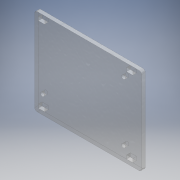
# Autodesk Inventor part: BBGW Case Bottom
Saved by Autodesk Inventor 2016 (Build 200138000, 138)
## iProperties
Created: 2016-06-26
Part Number: BBGW Case Bottom
Material: Acrylic, Clear
Document SubType Name: Modeling
Designer: Jacob
Density: 1.19 g/cm^3
Appearance: Transparent - Clear
Author: Jacob
Autodesk Inventor part; units mm, degrees
(part 1 of 2)
ref_plane "YZ Plane" through (0, 0, 0) normal (1, 0, 0) x (0, 1, 0)
ref_plane "XZ Plane" through (0, 0, 0) normal (0, 1, 0) x (-1, 0, 0)
ref_plane "XY Plane" through (0, 0, 0) normal (0, 0, 1) x (1, 0, 0)
sketch "Sketch1" plane through (0, 0, 0) normal (0, 1, 0) x (-1, 0, 0)
  line L0 (76.6427, 130.7252) -> (76.6428, 139.3252)
  spline S0 degree 3 poles (76.6428, 139.3252) (76.6428, 140.4298) (75.7473, 141.3252) (74.6428, 141.3252) knots 0 0 0 0 1 1 1 1
  line L1 (76.6428, 139.3252) -> (76.6428, 140.4298) construction
  line L2 (76.6428, 140.4298) -> (75.7473, 141.3252) construction
  line L3 (75.7473, 141.3252) -> (74.6428, 141.3252) construction
  line L4 (74.6428, 141.3252) -> (73.6427, 141.3252)
  line L5 (73.6427, 141.3252) -> (73.6427, 143.3252)
  line L6 (73.6427, 143.3252) -> (73.6422, 143.3593)
  line L7 (73.6422, 143.3593) -> (73.6404, 143.3934)
  line L8 (73.6404, 143.3934) -> (73.6375, 143.4275)
  line L9 (73.6375, 143.4275) -> (73.6334, 143.4614)
  line L10 (73.6334, 143.4614) -> (73.6282, 143.4951)
  line L11 (73.6282, 143.4951) -> (73.6218, 143.5287)
  line L12 (73.6218, 143.5287) -> (73.6143, 143.562)
  line L13 (73.6143, 143.562) -> (73.6057, 143.595)
  line L14 (73.6057, 143.595) -> (73.5959, 143.6277)
  line L15 (73.5959, 143.6277) -> (73.585, 143.6601)
  line L16 (73.585, 143.6601) -> (73.573, 143.6921)
  line L17 (73.573, 143.6921) -> (73.56, 143.7236)
  line L18 (73.56, 143.7236) -> (73.5458, 143.7547)
  line L19 (73.5458, 143.7547) -> (73.5306, 143.7853)
  line L20 (73.5306, 143.7853) -> (73.5144, 143.8153)
  line L21 (73.5144, 143.8153) -> (73.4972, 143.8448)
  line L22 (73.4972, 143.8448) -> (73.4789, 143.8737)
  line L23 (73.4789, 143.8737) -> (73.4597, 143.9019)
  line L24 (73.4597, 143.9019) -> (73.4396, 143.9294)
  line L25 (73.4396, 143.9294) -> (73.4185, 143.9563)
  line L26 (73.4185, 143.9563) -> (73.3965, 143.9824)
  line L27 (73.3965, 143.9824) -> (73.3736, 144.0078)
  line L28 (73.3736, 144.0078) -> (73.3499, 144.0323)
  line L29 (73.3499, 144.0323) -> (73.3253, 144.056)
  line L30 (73.3253, 144.056) -> (73.3, 144.0789)
  line L31 (73.3, 144.0789) -> (73.2738, 144.1009)
  line L32 (73.2738, 144.1009) -> (73.247, 144.122)
  line L33 (73.247, 144.122) -> (73.2194, 144.1422)
  line L34 (73.2194, 144.1422) -> (73.1912, 144.1614)
  line L35 (73.1912, 144.1614) -> (73.1623, 144.1796)
  line L36 (73.1623, 144.1796) -> (73.1329, 144.1969)
  line L37 (73.1329, 144.1969) -> (73.1028, 144.2131)
  line L38 (73.1028, 144.2131) -> (73.0722, 144.2283)
  line L39 (73.0722, 144.2283) -> (73.0412, 144.2424)
  line L40 (73.0412, 144.2424) -> (73.0096, 144.2555)
  line L41 (73.0096, 144.2555) -> (72.9776, 144.2675)
  line L42 (72.9776, 144.2675) -> (72.9453, 144.2783)
  line L43 (72.9453, 144.2783) -> (72.9125, 144.2881)
  line L44 (72.9125, 144.2881) -> (72.8795, 144.2968)
  line L45 (72.8795, 144.2968) -> (72.8462, 144.3043)
  line L46 (72.8462, 144.3043) -> (72.8127, 144.3107)
  line L47 (72.8127, 144.3107) -> (72.7789, 144.3159)
  line L48 (72.7789, 144.3159) -> (72.745, 144.32)
  line L49 (72.745, 144.32) -> (72.711, 144.3229)
  line L50 (72.711, 144.3229) -> (72.6769, 144.3246)
  line L51 (72.6769, 144.3246) -> (72.6428, 144.3252)
  line L52 (72.6428, 144.3252) -> (69.6427, 144.3252)
  line L53 (69.6427, 144.3252) -> (69.6086, 144.3246)
  line L54 (69.6086, 144.3246) -> (69.5745, 144.3229)
  line L55 (69.5745, 144.3229) -> (69.5405, 144.32)
  line L56 (69.5405, 144.32) -> (69.5066, 144.3159)
  line L57 (69.5066, 144.3159) -> (69.4728, 144.3107)
  line L58 (69.4728, 144.3107) -> (69.4393, 144.3043)
  line L59 (69.4393, 144.3043) -> (69.406, 144.2968)
  line L60 (69.406, 144.2968) -> (69.373, 144.2881)
  line L61 (69.373, 144.2881) -> (69.3402, 144.2783)
  line L62 (69.3402, 144.2783) -> (69.3079, 144.2675)
  line L63 (69.3079, 144.2675) -> (69.2759, 144.2555)
  line L64 (69.2759, 144.2555) -> (69.2443, 144.2424)
  line L65 (69.2443, 144.2424) -> (69.2133, 144.2283)
  line L66 (69.2133, 144.2283) -> (69.1827, 144.2131)
  line L67 (69.1827, 144.2131) -> (69.1526, 144.1969)
  line L68 (69.1526, 144.1969) -> (69.1232, 144.1796)
  line L69 (69.1232, 144.1796) -> (69.0943, 144.1614)
  line L70 (69.0943, 144.1614) -> (69.0661, 144.1422)
  line L71 (69.0661, 144.1422) -> (69.0385, 144.122)
  line L72 (69.0385, 144.122) -> (69.0117, 144.1009)
  line L73 (69.0117, 144.1009) -> (68.9855, 144.0789)
  line L74 (68.9855, 144.0789) -> (68.9602, 144.056)
  line L75 (68.9602, 144.056) -> (68.9356, 144.0323)
  line L76 (68.9356, 144.0323) -> (68.9119, 144.0078)
  line L77 (68.9119, 144.0078) -> (68.889, 143.9824)
  line L78 (68.889, 143.9824) -> (68.867, 143.9563)
  line L79 (68.867, 143.9563) -> (68.8459, 143.9294)
  line L80 (68.8459, 143.9294) -> (68.8258, 143.9019)
  line L81 (68.8258, 143.9019) -> (68.8066, 143.8737)
  line L82 (68.8066, 143.8737) -> (68.7883, 143.8448)
  line L83 (68.7883, 143.8448) -> (68.7711, 143.8153)
  line L84 (68.7711, 143.8153) -> (68.7549, 143.7853)
  line L85 (68.7549, 143.7853) -> (68.7397, 143.7547)
  line L86 (68.7397, 143.7547) -> (68.7255, 143.7236)
  line L87 (68.7255, 143.7236) -> (68.7125, 143.6921)
  line L88 (68.7125, 143.6921) -> (68.7005, 143.6601)
  line L89 (68.7005, 143.6601) -> (68.6896, 143.6277)
  line L90 (68.6896, 143.6277) -> (68.6798, 143.595)
  line L91 (68.6798, 143.595) -> (68.6712, 143.562)
  line L92 (68.6712, 143.562) -> (68.6637, 143.5287)
  line L93 (68.6637, 143.5287) -> (68.6573, 143.4951)
  line L94 (68.6573, 143.4951) -> (68.6521, 143.4614)
  line L95 (68.6521, 143.4614) -> (68.648, 143.4275)
  line L96 (68.648, 143.4275) -> (68.6451, 143.3934)
  line L97 (68.6451, 143.3934) -> (68.6433, 143.3593)
  line L98 (68.6433, 143.3593) -> (68.6427, 143.3252)
  line L99 (68.6427, 143.3252) -> (68.6427, 141.3252)
  line L100 (68.6427, 141.3252) -> (1.8263, 141.3252)
  line L101 (1.8263, 141.3252) -> (1.8263, 143.3252)
  line L102 (1.8263, 143.3252) -> (1.8258, 143.3593)
  line L103 (1.8258, 143.3593) -> (1.824, 143.3934)
  line L104 (1.824, 143.3934) -> (1.8211, 143.4275)
  line L105 (1.8211, 143.4275) -> (1.817, 143.4614)
  line L106 (1.817, 143.4614) -> (1.8118, 143.4951)
  line L107 (1.8118, 143.4951) -> (1.8054, 143.5287)
  line L108 (1.8054, 143.5287) -> (1.7979, 143.562)
  line L109 (1.7979, 143.562) -> (1.7893, 143.595)
  line L110 (1.7893, 143.595) -> (1.7795, 143.6277)
  line L111 (1.7795, 143.6277) -> (1.7686, 143.6601)
  line L112 (1.7686, 143.6601) -> (1.7566, 143.6921)
  line L113 (1.7566, 143.6921) -> (1.7436, 143.7236)
  line L114 (1.7436, 143.7236) -> (1.7294, 143.7547)
  line L115 (1.7294, 143.7547) -> (1.7142, 143.7853)
  line L116 (1.7142, 143.7853) -> (1.698, 143.8153)
  line L117 (1.698, 143.8153) -> (1.6808, 143.8448)
  line L118 (1.6808, 143.8448) -> (1.6625, 143.8737)
  line L119 (1.6625, 143.8737) -> (1.6433, 143.9019)
  line L120 (1.6433, 143.9019) -> (1.6231, 143.9294)
  line L121 (1.6231, 143.9294) -> (1.6021, 143.9563)
  line L122 (1.6021, 143.9563) -> (1.5801, 143.9824)
  line L123 (1.5801, 143.9824) -> (1.5572, 144.0078)
  line L124 (1.5572, 144.0078) -> (1.5334, 144.0323)
  line L125 (1.5334, 144.0323) -> (1.5089, 144.056)
  line L126 (1.5089, 144.056) -> (1.4835, 144.0789)
  line L127 (1.4835, 144.0789) -> (1.4574, 144.1009)
  line L128 (1.4574, 144.1009) -> (1.4306, 144.122)
  line L129 (1.4306, 144.122) -> (1.403, 144.1422)
  line L130 (1.403, 144.1422) -> (1.3748, 144.1614)
  line L131 (1.3748, 144.1614) -> (1.3459, 144.1796)
  line L132 (1.3459, 144.1796) -> (1.3164, 144.1969)
  line L133 (1.3164, 144.1969) -> (1.2864, 144.2131)
  line L134 (1.2864, 144.2131) -> (1.2558, 144.2283)
  line L135 (1.2558, 144.2283) -> (1.2247, 144.2424)
  line L136 (1.2247, 144.2424) -> (1.1932, 144.2555)
  line L137 (1.1932, 144.2555) -> (1.1612, 144.2675)
  line L138 (1.1612, 144.2675) -> (1.1289, 144.2783)
  line L139 (1.1289, 144.2783) -> (1.0961, 144.2881)
  line L140 (1.0961, 144.2881) -> (1.0631, 144.2968)
  line L141 (1.0631, 144.2968) -> (1.0298, 144.3043)
  line L142 (1.0298, 144.3043) -> (0.9962, 144.3107)
  line L143 (0.9962, 144.3107) -> (0.9625, 144.3159)
  line L144 (0.9625, 144.3159) -> (0.9286, 144.32)
  line L145 (0.9286, 144.32) -> (0.8946, 144.3229)
  line L146 (0.8946, 144.3229) -> (0.8605, 144.3246)
  line L147 (0.8605, 144.3246) -> (0.8263, 144.3252)
  line L148 (0.8263, 144.3252) -> (-2.1737, 144.3252)
  line L149 (-2.1737, 144.3252) -> (-2.2078, 144.3246)
  line L150 (-2.2078, 144.3246) -> (-2.2419, 144.3229)
  line L151 (-2.2419, 144.3229) -> (-2.2759, 144.32)
  line L152 (-2.2759, 144.32) -> (-2.3098, 144.3159)
  line L153 (-2.3098, 144.3159) -> (-2.3436, 144.3107)
  line L154 (-2.3436, 144.3107) -> (-2.3771, 144.3043)
  line L155 (-2.3771, 144.3043) -> (-2.4104, 144.2968)
  line L156 (-2.4104, 144.2968) -> (-2.4435, 144.2881)
  line L157 (-2.4435, 144.2881) -> (-2.4762, 144.2783)
  line L158 (-2.4762, 144.2783) -> (-2.5085, 144.2675)
  line L159 (-2.5085, 144.2675) -> (-2.5405, 144.2555)
  line L160 (-2.5405, 144.2555) -> (-2.5721, 144.2424)
  line L161 (-2.5721, 144.2424) -> (-2.6031, 144.2283)
  line L162 (-2.6031, 144.2283) -> (-2.6337, 144.2131)
  line L163 (-2.6337, 144.2131) -> (-2.6638, 144.1969)
  line L164 (-2.6638, 144.1969) -> (-2.6932, 144.1796)
  line L165 (-2.6932, 144.1796) -> (-2.7221, 144.1614)
  line L166 (-2.7221, 144.1614) -> (-2.7503, 144.1422)
  line L167 (-2.7503, 144.1422) -> (-2.7779, 144.122)
  line L168 (-2.7779, 144.122) -> (-2.8047, 144.1009)
  line L169 (-2.8047, 144.1009) -> (-2.8309, 144.0789)
  line L170 (-2.8309, 144.0789) -> (-2.8562, 144.056)
  line L171 (-2.8562, 144.056) -> (-2.8808, 144.0323)
  line L172 (-2.8808, 144.0323) -> (-2.9045, 144.0078)
  line L173 (-2.9045, 144.0078) -> (-2.9274, 143.9824)
  line L174 (-2.9274, 143.9824) -> (-2.9494, 143.9563)
  line L175 (-2.9494, 143.9563) -> (-2.9705, 143.9294)
  line L176 (-2.9705, 143.9294) -> (-2.9906, 143.9019)
  line L177 (-2.9906, 143.9019) -> (-3.0098, 143.8737)
  line L178 (-3.0098, 143.8737) -> (-3.0281, 143.8448)
  line L179 (-3.0281, 143.8448) -> (-3.0453, 143.8153)
  line L180 (-3.0453, 143.8153) -> (-3.0615, 143.7853)
  line L181 (-3.0615, 143.7853) -> (-3.0767, 143.7547)
  line L182 (-3.0767, 143.7547) -> (-3.0909, 143.7236)
  line L183 (-3.0909, 143.7236) -> (-3.1039, 143.6921)
  line L184 (-3.1039, 143.6921) -> (-3.1159, 143.6601)
  line L185 (-3.1159, 143.6601) -> (-3.1268, 143.6277)
  line L186 (-3.1268, 143.6277) -> (-3.1366, 143.595)
  line L187 (-3.1366, 143.595) -> (-3.1452, 143.562)
  line L188 (-3.1452, 143.562) -> (-3.1527, 143.5287)
  line L189 (-3.1527, 143.5287) -> (-3.1591, 143.4951)
  line L190 (-3.1591, 143.4951) -> (-3.1643, 143.4614)
  line L191 (-3.1643, 143.4614) -> (-3.1684, 143.4275)
  line L192 (-3.1684, 143.4275) -> (-3.1713, 143.3934)
  line L193 (-3.1713, 143.3934) -> (-3.1731, 143.3593)
  line L194 (-3.1731, 143.3593) -> (-3.1737, 143.3252)
  line L195 (-3.1737, 143.3252) -> (-3.1737, 141.3252)
  line L196 (-3.1737, 141.3252) -> (-8.3571, 141.3252)
  spline S1 degree 3 poles (-8.3571, 141.3252) (-8.8876, 141.3252) (-9.3963, 141.1145) (-9.7714, 140.7394) knots 0 0 0 0 0.5 0.5 0.5 0.5
  line L197 (-8.3571, 141.3252) -> (-8.8876, 141.3252) construction
  line L198 (-8.8876, 141.3252) -> (-9.3963, 141.1145) construction
  line L199 (-9.3963, 141.1145) -> (-9.7714, 140.7394) construction
  spline S2 degree 3 poles (-9.7714, 140.7394) (-9.771775, 140.739025) (-10.1464, 140.3643) (-10.3571, 139.8556) (-10.3571, 139.3252) knots 0.5 0.5 0.5 0.5 0.50000001 1 1 1 1
  line L200 (-9.7714, 140.7394) -> (-9.7714, 140.7394) construction
  line L201 (-9.7714, 140.7394) -> (-10.1464, 140.3643) construction
  line L202 (-10.1464, 140.3643) -> (-10.3571, 139.8556) construction
  line L203 (-10.3571, 139.8556) -> (-10.3571, 139.3252) construction
  line L204 (-10.3571, 139.3252) -> (-10.3572, 130.7252)
  spline S3 degree 3 poles (-10.3572, 130.7252) (-10.3572, 130.1948) (-10.1464, 129.6861) (-9.7714, 129.311) knots 0 0 0 0 0.5 0.5 0.5 0.5
  line L205 (-10.3572, 130.7252) -> (-10.3572, 130.1948) construction
  line L206 (-10.3572, 130.1948) -> (-10.1464, 129.6861) construction
  line L207 (-10.1464, 129.6861) -> (-9.7714, 129.311) construction
  spline S4 degree 3 poles (-9.7714, 129.311) (-9.771025, 129.310625) (-9.3963, 128.9359) (-8.8876, 128.7252) (-8.3572, 128.7252) knots 0.5 0.5 0.5 0.5 0.50000001 1 1 1 1
  line L208 (-9.7714, 129.311) -> (-9.7714, 129.311) construction
  line L209 (-9.7714, 129.311) -> (-9.3963, 128.9359) construction
  line L210 (-9.3963, 128.9359) -> (-8.8876, 128.7252) construction
  line L211 (-8.8876, 128.7252) -> (-8.3572, 128.7252) construction
  line L212 (-8.3572, 128.7252) -> (-3.1737, 128.7252)
  line L213 (-3.1737, 128.7252) -> (-3.1737, 126.7252)
  line L214 (-3.1737, 126.7252) -> (-3.1731, 126.6911)
  line L215 (-3.1731, 126.6911) -> (-3.1713, 126.657)
  line L216 (-3.1713, 126.657) -> (-3.1684, 126.6229)
  line L217 (-3.1684, 126.6229) -> (-3.1643, 126.589)
  line L218 (-3.1643, 126.589) -> (-3.1591, 126.5553)
  line L219 (-3.1591, 126.5553) -> (-3.1527, 126.5217)
  line L220 (-3.1527, 126.5217) -> (-3.1452, 126.4884)
  line L221 (-3.1452, 126.4884) -> (-3.1366, 126.4554)
  line L222 (-3.1366, 126.4554) -> (-3.1268, 126.4227)
  line L223 (-3.1268, 126.4227) -> (-3.1159, 126.3903)
  line L224 (-3.1159, 126.3903) -> (-3.1039, 126.3583)
  line L225 (-3.1039, 126.3583) -> (-3.0909, 126.3268)
  line L226 (-3.0909, 126.3268) -> (-3.0767, 126.2957)
  line L227 (-3.0767, 126.2957) -> (-3.0615, 126.2651)
  line L228 (-3.0615, 126.2651) -> (-3.0453, 126.2351)
  line L229 (-3.0453, 126.2351) -> (-3.0281, 126.2056)
  line L230 (-3.0281, 126.2056) -> (-3.0098, 126.1767)
  line L231 (-3.0098, 126.1767) -> (-2.9906, 126.1485)
  line L232 (-2.9906, 126.1485) -> (-2.9705, 126.121)
  line L233 (-2.9705, 126.121) -> (-2.9494, 126.0941)
  line L234 (-2.9494, 126.0941) -> (-2.9274, 126.068)
  line L235 (-2.9274, 126.068) -> (-2.9045, 126.0426)
  line L236 (-2.9045, 126.0426) -> (-2.8808, 126.0181)
  line L237 (-2.8808, 126.0181) -> (-2.8562, 125.9944)
  line L238 (-2.8562, 125.9944) -> (-2.8309, 125.9715)
  line L239 (-2.8309, 125.9715) -> (-2.8047, 125.9495)
  line L240 (-2.8047, 125.9495) -> (-2.7779, 125.9284)
  line L241 (-2.7779, 125.9284) -> (-2.7503, 125.9082)
  line L242 (-2.7503, 125.9082) -> (-2.7221, 125.889)
  line L243 (-2.7221, 125.889) -> (-2.6932, 125.8708)
  line L244 (-2.6932, 125.8708) -> (-2.6638, 125.8535)
  line L245 (-2.6638, 125.8535) -> (-2.6337, 125.8373)
  line L246 (-2.6337, 125.8373) -> (-2.6031, 125.8221)
  line L247 (-2.6031, 125.8221) -> (-2.5721, 125.808)
  line L248 (-2.5721, 125.808) -> (-2.5405, 125.7949)
  line L249 (-2.5405, 125.7949) -> (-2.5085, 125.7829)
  line L250 (-2.5085, 125.7829) -> (-2.4762, 125.7721)
  line L251 (-2.4762, 125.7721) -> (-2.4435, 125.7623)
  line L252 (-2.4435, 125.7623) -> (-2.4104, 125.7536)
  line L253 (-2.4104, 125.7536) -> (-2.3771, 125.7461)
  line L254 (-2.3771, 125.7461) -> (-2.3436, 125.7397)
  line L255 (-2.3436, 125.7397) -> (-2.3098, 125.7345)
  line L256 (-2.3098, 125.7345) -> (-2.2759, 125.7304)
  line L257 (-2.2759, 125.7304) -> (-2.2419, 125.7275)
  line L258 (-2.2419, 125.7275) -> (-2.2078, 125.7258)
  line L259 (-2.2078, 125.7258) -> (-2.1737, 125.7252)
  line L260 (-2.1737, 125.7252) -> (0.8263, 125.7252)
  line L261 (0.8263, 125.7252) -> (0.8605, 125.7258)
  line L262 (0.8605, 125.7258) -> (0.8946, 125.7275)
  line L263 (0.8946, 125.7275) -> (0.9286, 125.7304)
  line L264 (0.9286, 125.7304) -> (0.9625, 125.7345)
  line L265 (0.9625, 125.7345) -> (0.9962, 125.7397)
  line L266 (0.9962, 125.7397) -> (1.0298, 125.7461)
  line L267 (1.0298, 125.7461) -> (1.0631, 125.7536)
  line L268 (1.0631, 125.7536) -> (1.0961, 125.7623)
  line L269 (1.0961, 125.7623) -> (1.1289, 125.7721)
  line L270 (1.1289, 125.7721) -> (1.1612, 125.7829)
  line L271 (1.1612, 125.7829) -> (1.1932, 125.7949)
  line L272 (1.1932, 125.7949) -> (1.2247, 125.808)
  line L273 (1.2247, 125.808) -> (1.2558, 125.8221)
  line L274 (1.2558, 125.8221) -> (1.2864, 125.8373)
  line L275 (1.2864, 125.8373) -> (1.3164, 125.8535)
  line L276 (1.3164, 125.8535) -> (1.3459, 125.8708)
  line L277 (1.3459, 125.8708) -> (1.3748, 125.889)
  line L278 (1.3748, 125.889) -> (1.403, 125.9082)
  line L279 (1.403, 125.9082) -> (1.4306, 125.9284)
  line L280 (1.4306, 125.9284) -> (1.4574, 125.9495)
  line L281 (1.4574, 125.9495) -> (1.4835, 125.9715)
  line L282 (1.4835, 125.9715) -> (1.5089, 125.9944)
  line L283 (1.5089, 125.9944) -> (1.5334, 126.0181)
  line L284 (1.5334, 126.0181) -> (1.5572, 126.0426)
  line L285 (1.5572, 126.0426) -> (1.5801, 126.068)
  line L286 (1.5801, 126.068) -> (1.6021, 126.0941)
  line L287 (1.6021, 126.0941) -> (1.6231, 126.121)
  line L288 (1.6231, 126.121) -> (1.6433, 126.1485)
  line L289 (1.6433, 126.1485) -> (1.6625, 126.1767)
  line L290 (1.6625, 126.1767) -> (1.6808, 126.2056)
  line L291 (1.6808, 126.2056) -> (1.698, 126.2351)
  line L292 (1.698, 126.2351) -> (1.7142, 126.2651)
  line L293 (1.7142, 126.2651) -> (1.7294, 126.2957)
  line L294 (1.7294, 126.2957) -> (1.7436, 126.3268)
  line L295 (1.7436, 126.3268) -> (1.7566, 126.3583)
  line L296 (1.7566, 126.3583) -> (1.7686, 126.3903)
  line L297 (1.7686, 126.3903) -> (1.7795, 126.4227)
  line L298 (1.7795, 126.4227) -> (1.7893, 126.4554)
  line L299 (1.7893, 126.4554) -> (1.7979, 126.4884)
  line L300 (1.7979, 126.4884) -> (1.8054, 126.5217)
  line L301 (1.8054, 126.5217) -> (1.8118, 126.5553)
  line L302 (1.8118, 126.5553) -> (1.817, 126.589)
  line L303 (1.817, 126.589) -> (1.8211, 126.6229)
  line L304 (1.8211, 126.6229) -> (1.824, 126.657)
  line L305 (1.824, 126.657) -> (1.8258, 126.6911)
  line L306 (1.8258, 126.6911) -> (1.8263, 126.7252)
  line L307 (1.8263, 126.7252) -> (1.8263, 128.7252)
  line L308 (1.8263, 128.7252) -> (68.6427, 128.7252)
  line L309 (68.6427, 128.7252) -> (68.6427, 126.7252)
  line L310 (68.6427, 126.7252) -> (68.6433, 126.6911)
  line L311 (68.6433, 126.6911) -> (68.6451, 126.657)
  line L312 (68.6451, 126.657) -> (68.648, 126.6229)
  line L313 (68.648, 126.6229) -> (68.6521, 126.589)
  line L314 (68.6521, 126.589) -> (68.6573, 126.5553)
  line L315 (68.6573, 126.5553) -> (68.6637, 126.5217)
  line L316 (68.6637, 126.5217) -> (68.6712, 126.4884)
  line L317 (68.6712, 126.4884) -> (68.6798, 126.4554)
  line L318 (68.6798, 126.4554) -> (68.6896, 126.4227)
  line L319 (68.6896, 126.4227) -> (68.7005, 126.3903)
  line L320 (68.7005, 126.3903) -> (68.7125, 126.3583)
  line L321 (68.7125, 126.3583) -> (68.7255, 126.3268)
  line L322 (68.7255, 126.3268) -> (68.7397, 126.2957)
  line L323 (68.7397, 126.2957) -> (68.7549, 126.2651)
  line L324 (68.7549, 126.2651) -> (68.7711, 126.2351)
  line L325 (68.7711, 126.2351) -> (68.7883, 126.2056)
  line L326 (68.7883, 126.2056) -> (68.8066, 126.1767)
  line L327 (68.8066, 126.1767) -> (68.8258, 126.1485)
  line L328 (68.8258, 126.1485) -> (68.8459, 126.121)
  line L329 (68.8459, 126.121) -> (68.867, 126.0941)
  line L330 (68.867, 126.0941) -> (68.889, 126.068)
  line L331 (68.889, 126.068) -> (68.9119, 126.0426)
  line L332 (68.9119, 126.0426) -> (68.9356, 126.0181)
  line L333 (68.9356, 126.0181) -> (68.9602, 125.9944)
  line L334 (68.9602, 125.9944) -> (68.9855, 125.9715)
  line L335 (68.9855, 125.9715) -> (69.0117, 125.9495)
  line L336 (69.0117, 125.9495) -> (69.0385, 125.9284)
  line L337 (69.0385, 125.9284) -> (69.0661, 125.9082)
  line L338 (69.0661, 125.9082) -> (69.0943, 125.889)
  line L339 (69.0943, 125.889) -> (69.1232, 125.8708)
  line L340 (69.1232, 125.8708) -> (69.1526, 125.8535)
  line L341 (69.1526, 125.8535) -> (69.1827, 125.8373)
  line L342 (69.1827, 125.8373) -> (69.2133, 125.8221)
  line L343 (69.2133, 125.8221) -> (69.2443, 125.808)
  line L344 (69.2443, 125.808) -> (69.2759, 125.7949)
  line L345 (69.2759, 125.7949) -> (69.3079, 125.7829)
  line L346 (69.3079, 125.7829) -> (69.3402, 125.7721)
  line L347 (69.3402, 125.7721) -> (69.373, 125.7623)
  line L348 (69.373, 125.7623) -> (69.406, 125.7536)
  line L349 (69.406, 125.7536) -> (69.4393, 125.7461)
  line L350 (69.4393, 125.7461) -> (69.4728, 125.7397)
  line L351 (69.4728, 125.7397) -> (69.5066, 125.7345)
  line L352 (69.5066, 125.7345) -> (69.5405, 125.7304)
  line L353 (69.5405, 125.7304) -> (69.5745, 125.7275)
  line L354 (69.5745, 125.7275) -> (69.6086, 125.7258)
  line L355 (69.6086, 125.7258) -> (69.6427, 125.7252)
  line L356 (69.6427, 125.7252) -> (72.6428, 125.7252)
  line L357 (72.6428, 125.7252) -> (72.6769, 125.7258)
  line L358 (72.6769, 125.7258) -> (72.711, 125.7275)
  line L359 (72.711, 125.7275) -> (72.745, 125.7304)
  line L360 (72.745, 125.7304) -> (72.7789, 125.7345)
  line L361 (72.7789, 125.7345) -> (72.8127, 125.7397)
  line L362 (72.8127, 125.7397) -> (72.8462, 125.7461)
  line L363 (72.8462, 125.7461) -> (72.8795, 125.7536)
  line L364 (72.8795, 125.7536) -> (72.9125, 125.7623)
  line L365 (72.9125, 125.7623) -> (72.9453, 125.7721)
  line L366 (72.9453, 125.7721) -> (72.9776, 125.7829)
  line L367 (72.9776, 125.7829) -> (73.0096, 125.7949)
  line L368 (73.0096, 125.7949) -> (73.0412, 125.808)
  line L369 (73.0412, 125.808) -> (73.0722, 125.8221)
  line L370 (73.0722, 125.8221) -> (73.1028, 125.8373)
  line L371 (73.1028, 125.8373) -> (73.1329, 125.8535)
  line L372 (73.1329, 125.8535) -> (73.1623, 125.8708)
  line L373 (73.1623, 125.8708) -> (73.1912, 125.889)
  line L374 (73.1912, 125.889) -> (73.2194, 125.9082)
  line L375 (73.2194, 125.9082) -> (73.247, 125.9284)
  line L376 (73.247, 125.9284) -> (73.2738, 125.9495)
  line L377 (73.2738, 125.9495) -> (73.3, 125.9715)
  line L378 (73.3, 125.9715) -> (73.3253, 125.9944)
  line L379 (73.3253, 125.9944) -> (73.3499, 126.0181)
  line L380 (73.3499, 126.0181) -> (73.3736, 126.0426)
  line L381 (73.3736, 126.0426) -> (73.3965, 126.068)
  line L382 (73.3965, 126.068) -> (73.4185, 126.0941)
  line L383 (73.4185, 126.0941) -> (73.4396, 126.121)
  line L384 (73.4396, 126.121) -> (73.4597, 126.1485)
  line L385 (73.4597, 126.1485) -> (73.4789, 126.1767)
  line L386 (73.4789, 126.1767) -> (73.4972, 126.2056)
  line L387 (73.4972, 126.2056) -> (73.5144, 126.2351)
  line L388 (73.5144, 126.2351) -> (73.5306, 126.2651)
  line L389 (73.5306, 126.2651) -> (73.5458, 126.2957)
  line L390 (73.5458, 126.2957) -> (73.56, 126.3268)
  line L391 (73.56, 126.3268) -> (73.573, 126.3583)
  line L392 (73.573, 126.3583) -> (73.585, 126.3903)
  line L393 (73.585, 126.3903) -> (73.5959, 126.4227)
  line L394 (73.5959, 126.4227) -> (73.6057, 126.4554)
  line L395 (73.6057, 126.4554) -> (73.6143, 126.4884)
  line L396 (73.6143, 126.4884) -> (73.6218, 126.5217)
  line L397 (73.6218, 126.5217) -> (73.6282, 126.5553)
  line L398 (73.6282, 126.5553) -> (73.6334, 126.589)
  line L399 (73.6334, 126.589) -> (73.6375, 126.6229)
  line L400 (73.6375, 126.6229) -> (73.6404, 126.657)
  line L401 (73.6404, 126.657) -> (73.6422, 126.6911)
  line L402 (73.6422, 126.6911) -> (73.6428, 126.7252)
  line L403 (73.6428, 126.7252) -> (73.6427, 128.7252)
  line L404 (73.6427, 128.7252) -> (74.6427, 128.7252)
  spline S5 degree 3 poles (74.6428, 128.7252) (75.7473, 128.7252) (76.6427, 129.6206) (76.6427, 130.7252) knots 0 0 0 0 1 1 1 1
  line L405 (74.6428, 128.7252) -> (75.7473, 128.7252) construction
  line L406 (75.7473, 128.7252) -> (76.6427, 129.6206) construction
  line L407 (76.6427, 129.6206) -> (76.6427, 130.7252) construction
  line L408 (-13.3571, 130.7252) -> (-13.357, 139.3252)
  spline S6 degree 3 poles (-13.357, 139.3252) (-13.357, 140.4298) (-14.2525, 141.3252) (-15.357, 141.3252) knots 0 0 0 0 1 1 1 1
  line L409 (-13.357, 139.3252) -> (-13.357, 140.4298) construction
  line L410 (-13.357, 140.4298) -> (-14.2525, 141.3252) construction
  line L411 (-14.2525, 141.3252) -> (-15.357, 141.3252) construction
  line L412 (-15.357, 141.3252) -> (-16.3571, 141.3252)
  line L413 (-16.3571, 141.3252) -> (-16.3571, 143.3252)
  line L414 (-16.3571, 143.3252) -> (-16.3576, 143.3593)
  line L415 (-16.3576, 143.3593) -> (-16.3594, 143.3934)
  line L416 (-16.3594, 143.3934) -> (-16.3623, 143.4275)
  line L417 (-16.3623, 143.4275) -> (-16.3664, 143.4614)
  line L418 (-16.3664, 143.4614) -> (-16.3716, 143.4951)
  line L419 (-16.3716, 143.4951) -> (-16.378, 143.5287)
  line L420 (-16.378, 143.5287) -> (-16.3855, 143.562)
  line L421 (-16.3855, 143.562) -> (-16.3941, 143.595)
  line L422 (-16.3941, 143.595) -> (-16.4039, 143.6277)
  line L423 (-16.4039, 143.6277) -> (-16.4148, 143.6601)
  line L424 (-16.4148, 143.6601) -> (-16.4268, 143.6921)
  line L425 (-16.4268, 143.6921) -> (-16.4398, 143.7236)
  line L426 (-16.4398, 143.7236) -> (-16.454, 143.7547)
  line L427 (-16.454, 143.7547) -> (-16.4692, 143.7853)
  line L428 (-16.4692, 143.7853) -> (-16.4854, 143.8153)
  line L429 (-16.4854, 143.8153) -> (-16.5026, 143.8448)
  line L430 (-16.5026, 143.8448) -> (-16.5209, 143.8737)
  line L431 (-16.5209, 143.8737) -> (-16.5401, 143.9019)
  line L432 (-16.5401, 143.9019) -> (-16.5602, 143.9294)
  line L433 (-16.5602, 143.9294) -> (-16.5813, 143.9563)
  line L434 (-16.5813, 143.9563) -> (-16.6033, 143.9824)
  line L435 (-16.6033, 143.9824) -> (-16.6262, 144.0078)
  line L436 (-16.6262, 144.0078) -> (-16.6499, 144.0323)
  line L437 (-16.6499, 144.0323) -> (-16.6745, 144.056)
  line L438 (-16.6745, 144.056) -> (-16.6998, 144.0789)
  line L439 (-16.6998, 144.0789) -> (-16.726, 144.1009)
  line L440 (-16.726, 144.1009) -> (-16.7528, 144.122)
  line L441 (-16.7528, 144.122) -> (-16.7804, 144.1422)
  line L442 (-16.7804, 144.1422) -> (-16.8086, 144.1614)
  line L443 (-16.8086, 144.1614) -> (-16.8375, 144.1796)
  line L444 (-16.8375, 144.1796) -> (-16.8669, 144.1969)
  line L445 (-16.8669, 144.1969) -> (-16.897, 144.2131)
  line L446 (-16.897, 144.2131) -> (-16.9276, 144.2283)
  line L447 (-16.9276, 144.2283) -> (-16.9586, 144.2424)
  line L448 (-16.9586, 144.2424) -> (-16.9902, 144.2555)
  line L449 (-16.9902, 144.2555) -> (-17.0222, 144.2675)
  line L450 (-17.0222, 144.2675) -> (-17.0545, 144.2783)
  line L451 (-17.0545, 144.2783) -> (-17.0873, 144.2881)
  line L452 (-17.0873, 144.2881) -> (-17.1203, 144.2968)
  line L453 (-17.1203, 144.2968) -> (-17.1536, 144.3043)
  line L454 (-17.1536, 144.3043) -> (-17.1871, 144.3107)
  line L455 (-17.1871, 144.3107) -> (-17.2209, 144.3159)
  line L456 (-17.2209, 144.3159) -> (-17.2548, 144.32)
  line L457 (-17.2548, 144.32) -> (-17.2888, 144.3229)
  line L458 (-17.2888, 144.3229) -> (-17.3229, 144.3246)
  line L459 (-17.3229, 144.3246) -> (-17.3571, 144.3252)
  line L460 (-17.3571, 144.3252) -> (-20.3571, 144.3252)
  line L461 (-20.3571, 144.3252) -> (-20.3912, 144.3246)
  line L462 (-20.3912, 144.3246) -> (-20.4253, 144.3229)
  line L463 (-20.4253, 144.3229) -> (-20.4593, 144.32)
  line L464 (-20.4593, 144.32) -> (-20.4932, 144.3159)
  line L465 (-20.4932, 144.3159) -> (-20.527, 144.3107)
  line L466 (-20.527, 144.3107) -> (-20.5605, 144.3043)
  line L467 (-20.5605, 144.3043) -> (-20.5938, 144.2968)
  line L468 (-20.5938, 144.2968) -> (-20.6268, 144.2881)
  line L469 (-20.6268, 144.2881) -> (-20.6596, 144.2783)
  line L470 (-20.6596, 144.2783) -> (-20.6919, 144.2675)
  line L471 (-20.6919, 144.2675) -> (-20.7239, 144.2555)
  line L472 (-20.7239, 144.2555) -> (-20.7555, 144.2424)
  line L473 (-20.7555, 144.2424) -> (-20.7865, 144.2283)
  line L474 (-20.7865, 144.2283) -> (-20.8171, 144.2131)
  line L475 (-20.8171, 144.2131) -> (-20.8472, 144.1969)
  line L476 (-20.8472, 144.1969) -> (-20.8766, 144.1796)
  line L477 (-20.8766, 144.1796) -> (-20.9055, 144.1614)
  line L478 (-20.9055, 144.1614) -> (-20.9337, 144.1422)
  line L479 (-20.9337, 144.1422) -> (-20.9613, 144.122)
  line L480 (-20.9613, 144.122) -> (-20.9881, 144.1009)
  line L481 (-20.9881, 144.1009) -> (-21.0143, 144.0789)
  line L482 (-21.0143, 144.0789) -> (-21.0396, 144.056)
  line L483 (-21.0396, 144.056) -> (-21.0642, 144.0323)
  line L484 (-21.0642, 144.0323) -> (-21.0879, 144.0078)
  line L485 (-21.0879, 144.0078) -> (-21.1108, 143.9824)
  line L486 (-21.1108, 143.9824) -> (-21.1328, 143.9563)
  line L487 (-21.1328, 143.9563) -> (-21.1539, 143.9294)
  line L488 (-21.1539, 143.9294) -> (-21.174, 143.9019)
  line L489 (-21.174, 143.9019) -> (-21.1932, 143.8737)
  line L490 (-21.1932, 143.8737) -> (-21.2115, 143.8448)
  line L491 (-21.2115, 143.8448) -> (-21.2287, 143.8153)
  line L492 (-21.2287, 143.8153) -> (-21.2449, 143.7853)
  line L493 (-21.2449, 143.7853) -> (-21.2601, 143.7547)
  line L494 (-21.2601, 143.7547) -> (-21.2743, 143.7236)
  line L495 (-21.2743, 143.7236) -> (-21.2873, 143.6921)
  line L496 (-21.2873, 143.6921) -> (-21.2993, 143.6601)
  line L497 (-21.2993, 143.6601) -> (-21.3102, 143.6277)
  line L498 (-21.3102, 143.6277) -> (-21.32, 143.595)
  line L499 (-21.32, 143.595) -> (-21.3286, 143.562)
  line L500 (-21.3286, 143.562) -> (-21.3361, 143.5287)
  line L501 (-21.3361, 143.5287) -> (-21.3425, 143.4951)
  line L502 (-21.3425, 143.4951) -> (-21.3477, 143.4614)
  line L503 (-21.3477, 143.4614) -> (-21.3518, 143.4275)
  line L504 (-21.3518, 143.4275) -> (-21.3547, 143.3934)
  line L505 (-21.3547, 143.3934) -> (-21.3565, 143.3593)
  line L506 (-21.3565, 143.3593) -> (-21.3571, 143.3252)
  line L507 (-21.3571, 143.3252) -> (-21.3571, 141.3252)
  line L508 (-21.3571, 141.3252) -> (-88.1735, 141.3252)
  line L509 (-88.1735, 141.3252) -> (-88.1735, 143.3252)
  line L510 (-88.1735, 143.3252) -> (-88.174, 143.3593)
  line L511 (-88.174, 143.3593) -> (-88.1758, 143.3934)
  line L512 (-88.1758, 143.3934) -> (-88.1787, 143.4275)
  line L513 (-88.1787, 143.4275) -> (-88.1828, 143.4614)
  line L514 (-88.1828, 143.4614) -> (-88.188, 143.4951)
  line L515 (-88.188, 143.4951) -> (-88.1944, 143.5287)
  line L516 (-88.1944, 143.5287) -> (-88.2019, 143.562)
  line L517 (-88.2019, 143.562) -> (-88.2105, 143.595)
  line L518 (-88.2105, 143.595) -> (-88.2203, 143.6277)
  line L519 (-88.2203, 143.6277) -> (-88.2312, 143.6601)
  line L520 (-88.2312, 143.6601) -> (-88.2432, 143.6921)
  line L521 (-88.2432, 143.6921) -> (-88.2562, 143.7236)
  line L522 (-88.2562, 143.7236) -> (-88.2704, 143.7547)
  line L523 (-88.2704, 143.7547) -> (-88.2856, 143.7853)
  line L524 (-88.2856, 143.7853) -> (-88.3018, 143.8153)
  line L525 (-88.3018, 143.8153) -> (-88.319, 143.8448)
  line L526 (-88.319, 143.8448) -> (-88.3373, 143.8737)
  line L527 (-88.3373, 143.8737) -> (-88.3565, 143.9019)
  line L528 (-88.3565, 143.9019) -> (-88.3767, 143.9294)
  line L529 (-88.3767, 143.9294) -> (-88.3977, 143.9563)
  line L530 (-88.3977, 143.9563) -> (-88.4197, 143.9824)
  line L531 (-88.4197, 143.9824) -> (-88.4426, 144.0078)
  line L532 (-88.4426, 144.0078) -> (-88.4664, 144.0323)
  line L533 (-88.4664, 144.0323) -> (-88.4909, 144.056)
  line L534 (-88.4909, 144.056) -> (-88.5163, 144.0789)
  line L535 (-88.5163, 144.0789) -> (-88.5424, 144.1009)
  line L536 (-88.5424, 144.1009) -> (-88.5692, 144.122)
  line L537 (-88.5692, 144.122) -> (-88.5968, 144.1422)
  line L538 (-88.5968, 144.1422) -> (-88.625, 144.1614)
  line L539 (-88.625, 144.1614) -> (-88.6539, 144.1796)
  line L540 (-88.6539, 144.1796) -> (-88.6834, 144.1969)
  line L541 (-88.6834, 144.1969) -> (-88.7134, 144.2131)
  line L542 (-88.7134, 144.2131) -> (-88.744, 144.2283)
  line L543 (-88.744, 144.2283) -> (-88.7751, 144.2424)
  line L544 (-88.7751, 144.2424) -> (-88.8066, 144.2555)
  line L545 (-88.8066, 144.2555) -> (-88.8386, 144.2675)
  line L546 (-88.8386, 144.2675) -> (-88.8709, 144.2783)
  line L547 (-88.8709, 144.2783) -> (-88.9037, 144.2881)
  line L548 (-88.9037, 144.2881) -> (-88.9367, 144.2968)
  line L549 (-88.9367, 144.2968) -> (-88.97, 144.3043)
  line L550 (-88.97, 144.3043) -> (-89.0036, 144.3107)
  line L551 (-89.0036, 144.3107) -> (-89.0373, 144.3159)
  line L552 (-89.0373, 144.3159) -> (-89.0712, 144.32)
  line L553 (-89.0712, 144.32) -> (-89.1052, 144.3229)
  line L554 (-89.1052, 144.3229) -> (-89.1393, 144.3246)
  line L555 (-89.1393, 144.3246) -> (-89.1735, 144.3252)
  line L556 (-89.1735, 144.3252) -> (-92.1735, 144.3252)
  line L557 (-92.1735, 144.3252) -> (-92.2076, 144.3246)
  line L558 (-92.2076, 144.3246) -> (-92.2417, 144.3229)
  line L559 (-92.2417, 144.3229) -> (-92.2757, 144.32)
  line L560 (-92.2757, 144.32) -> (-92.3096, 144.3159)
  line L561 (-92.3096, 144.3159) -> (-92.3434, 144.3107)
  line L562 (-92.3434, 144.3107) -> (-92.3769, 144.3043)
  line L563 (-92.3769, 144.3043) -> (-92.4102, 144.2968)
  line L564 (-92.4102, 144.2968) -> (-92.4433, 144.2881)
  line L565 (-92.4433, 144.2881) -> (-92.476, 144.2783)
  line L566 (-92.476, 144.2783) -> (-92.5083, 144.2675)
  line L567 (-92.5083, 144.2675) -> (-92.5403, 144.2555)
  line L568 (-92.5403, 144.2555) -> (-92.5719, 144.2424)
  line L569 (-92.5719, 144.2424) -> (-92.6029, 144.2283)
  line L570 (-92.6029, 144.2283) -> (-92.6335, 144.2131)
  line L571 (-92.6335, 144.2131) -> (-92.6636, 144.1969)
  line L572 (-92.6636, 144.1969) -> (-92.693, 144.1796)
  line L573 (-92.693, 144.1796) -> (-92.7219, 144.1614)
  line L574 (-92.7219, 144.1614) -> (-92.7501, 144.1422)
  line L575 (-92.7501, 144.1422) -> (-92.7777, 144.122)
  line L576 (-92.7777, 144.122) -> (-92.8045, 144.1009)
  line L577 (-92.8045, 144.1009) -> (-92.8307, 144.0789)
  line L578 (-92.8307, 144.0789) -> (-92.856, 144.056)
  line L579 (-92.856, 144.056) -> (-92.8806, 144.0323)
  line L580 (-92.8806, 144.0323) -> (-92.9043, 144.0078)
  line L581 (-92.9043, 144.0078) -> (-92.9272, 143.9824)
  line L582 (-92.9272, 143.9824) -> (-92.9492, 143.9563)
  line L583 (-92.9492, 143.9563) -> (-92.9703, 143.9294)
  line L584 (-92.9703, 143.9294) -> (-92.9904, 143.9019)
  line L585 (-92.9904, 143.9019) -> (-93.0096, 143.8737)
  line L586 (-93.0096, 143.8737) -> (-93.0279, 143.8448)
  line L587 (-93.0279, 143.8448) -> (-93.0451, 143.8153)
  line L588 (-93.0451, 143.8153) -> (-93.0613, 143.7853)
  line L589 (-93.0613, 143.7853) -> (-93.0765, 143.7547)
  line L590 (-93.0765, 143.7547) -> (-93.0907, 143.7236)
  line L591 (-93.0907, 143.7236) -> (-93.1037, 143.6921)
  line L592 (-93.1037, 143.6921) -> (-93.1157, 143.6601)
  line L593 (-93.1157, 143.6601) -> (-93.1266, 143.6277)
  line L594 (-93.1266, 143.6277) -> (-93.1364, 143.595)
  line L595 (-93.1364, 143.595) -> (-93.145, 143.562)
  line L596 (-93.145, 143.562) -> (-93.1525, 143.5287)
  line L597 (-93.1525, 143.5287) -> (-93.1589, 143.4951)
  line L598 (-93.1589, 143.4951) -> (-93.1641, 143.4614)
  line L599 (-93.1641, 143.4614) -> (-93.1682, 143.4275)
  line L600 (-93.1682, 143.4275) -> (-93.1711, 143.3934)
  line L601 (-93.1711, 143.3934) -> (-93.1729, 143.3593)
  line L602 (-93.1729, 143.3593) -> (-93.1735, 143.3252)
  line L603 (-93.1735, 143.3252) -> (-93.1735, 141.3252)
  line L604 (-93.1735, 141.3252) -> (-98.357, 141.3252)
  spline S7 degree 3 poles (-98.357, 141.3252) (-98.8875, 141.3252) (-99.3962, 141.1145) (-99.7713, 140.7394) knots 0 0 0 0 0.5 0.5 0.5 0.5
  line L605 (-98.357, 141.3252) -> (-98.8875, 141.3252) construction
  line L606 (-98.8875, 141.3252) -> (-99.3962, 141.1145) construction
  line L607 (-99.3962, 141.1145) -> (-99.7713, 140.7394) construction
  spline S8 degree 3 poles (-99.7713, 140.7394) (-99.771675, 140.739025) (-100.1463, 140.3643) (-100.357, 139.8556) (-100.357, 139.3252) knots 0.5 0.5 0.5 0.5 0.50000001 1 1 1 1
  line L608 (-99.7713, 140.7394) -> (-99.7713, 140.7394) construction
  line L609 (-99.7713, 140.7394) -> (-100.1463, 140.3643) construction
  line L610 (-100.1463, 140.3643) -> (-100.357, 139.8556) construction
  line L611 (-100.357, 139.8556) -> (-100.357, 139.3252) construction
  line L612 (-100.357, 139.3252) -> (-100.3571, 130.7252)
  spline S9 degree 3 poles (-100.3571, 130.7252) (-100.3571, 130.1948) (-100.1463, 129.6861) (-99.7713, 129.311) knots 0 0 0 0 0.5 0.5 0.5 0.5
  line L613 (-100.3571, 130.7252) -> (-100.3571, 130.1948) construction
  line L614 (-100.3571, 130.1948) -> (-100.1463, 129.6861) construction
  line L615 (-100.1463, 129.6861) -> (-99.7713, 129.311) construction
  spline S10 degree 3 poles (-99.7713, 129.311) (-99.770925, 129.310625) (-99.3962, 128.9359) (-98.8875, 128.7252) (-98.3571, 128.7252) knots 0.5 0.5 0.5 0.5 0.50000001 1 1 1 1
  line L616 (-99.7713, 129.311) -> (-99.7713, 129.311) construction
  line L617 (-99.7713, 129.311) -> (-99.3962, 128.9359) construction
  line L618 (-99.3962, 128.9359) -> (-98.8875, 128.7252) construction
  line L619 (-98.8875, 128.7252) -> (-98.3571, 128.7252) construction
  line L620 (-98.3571, 128.7252) -> (-93.1735, 128.7252)
  line L621 (-93.1735, 128.7252) -> (-93.1735, 126.7252)
  line L622 (-93.1735, 126.7252) -> (-93.1729, 126.6911)
  line L623 (-93.1729, 126.6911) -> (-93.1711, 126.657)
  line L624 (-93.1711, 126.657) -> (-93.1682, 126.6229)
  line L625 (-93.1682, 126.6229) -> (-93.1641, 126.589)
  line L626 (-93.1641, 126.589) -> (-93.1589, 126.5553)
  line L627 (-93.1589, 126.5553) -> (-93.1525, 126.5217)
  line L628 (-93.1525, 126.5217) -> (-93.145, 126.4884)
  line L629 (-93.145, 126.4884) -> (-93.1364, 126.4554)
  line L630 (-93.1364, 126.4554) -> (-93.1266, 126.4227)
  line L631 (-93.1266, 126.4227) -> (-93.1157, 126.3903)
  line L632 (-93.1157, 126.3903) -> (-93.1037, 126.3583)
  line L633 (-93.1037, 126.3583) -> (-93.0907, 126.3268)
  line L634 (-93.0907, 126.3268) -> (-93.0765, 126.2957)
  line L635 (-93.0765, 126.2957) -> (-93.0613, 126.2651)
  line L636 (-93.0613, 126.2651) -> (-93.0451, 126.2351)
  line L637 (-93.0451, 126.2351) -> (-93.0279, 126.2056)
  line L638 (-93.0279, 126.2056) -> (-93.0096, 126.1767)
  line L639 (-93.0096, 126.1767) -> (-92.9904, 126.1485)
  line L640 (-92.9904, 126.1485) -> (-92.9703, 126.121)
  line L641 (-92.9703, 126.121) -> (-92.9492, 126.0941)
  line L642 (-92.9492, 126.0941) -> (-92.9272, 126.068)
  line L643 (-92.9272, 126.068) -> (-92.9043, 126.0426)
  line L644 (-92.9043, 126.0426) -> (-92.8806, 126.0181)
  line L645 (-92.8806, 126.0181) -> (-92.856, 125.9944)
  line L646 (-92.856, 125.9944) -> (-92.8307, 125.9715)
  line L647 (-92.8307, 125.9715) -> (-92.8045, 125.9495)
  line L648 (-92.8045, 125.9495) -> (-92.7777, 125.9284)
  line L649 (-92.7777, 125.9284) -> (-92.7501, 125.9082)
  line L650 (-92.7501, 125.9082) -> (-92.7219, 125.889)
  line L651 (-92.7219, 125.889) -> (-92.693, 125.8708)
  line L652 (-92.693, 125.8708) -> (-92.6636, 125.8535)
  line L653 (-92.6636, 125.8535) -> (-92.6335, 125.8373)
  line L654 (-92.6335, 125.8373) -> (-92.6029, 125.8221)
  line L655 (-92.6029, 125.8221) -> (-92.5719, 125.808)
  line L656 (-92.5719, 125.808) -> (-92.5403, 125.7949)
  line L657 (-92.5403, 125.7949) -> (-92.5083, 125.7829)
  line L658 (-92.5083, 125.7829) -> (-92.476, 125.7721)
  line L659 (-92.476, 125.7721) -> (-92.4433, 125.7623)
  line L660 (-92.4433, 125.7623) -> (-92.4102, 125.7536)
  line L661 (-92.4102, 125.7536) -> (-92.3769, 125.7461)
  line L662 (-92.3769, 125.7461) -> (-92.3434, 125.7397)
  line L663 (-92.3434, 125.7397) -> (-92.3096, 125.7345)
  line L664 (-92.3096, 125.7345) -> (-92.2757, 125.7304)
  line L665 (-92.2757, 125.7304) -> (-92.2417, 125.7275)
  line L666 (-92.2417, 125.7275) -> (-92.2076, 125.7258)
  line L667 (-92.2076, 125.7258) -> (-92.1735, 125.7252)
  line L668 (-92.1735, 125.7252) -> (-89.1735, 125.7252)
  line L669 (-89.1735, 125.7252) -> (-89.1393, 125.7258)
  line L670 (-89.1393, 125.7258) -> (-89.1052, 125.7275)
  line L671 (-89.1052, 125.7275) -> (-89.0712, 125.7304)
  line L672 (-89.0712, 125.7304) -> (-89.0373, 125.7345)
  line L673 (-89.0373, 125.7345) -> (-89.0036, 125.7397)
  line L674 (-89.0036, 125.7397) -> (-88.97, 125.7461)
  line L675 (-88.97, 125.7461) -> (-88.9367, 125.7536)
  line L676 (-88.9367, 125.7536) -> (-88.9037, 125.7623)
  line L677 (-88.9037, 125.7623) -> (-88.8709, 125.7721)
  line L678 (-88.8709, 125.7721) -> (-88.8386, 125.7829)
  line L679 (-88.8386, 125.7829) -> (-88.8066, 125.7949)
  line L680 (-88.8066, 125.7949) -> (-88.7751, 125.808)
  line L681 (-88.7751, 125.808) -> (-88.744, 125.8221)
  line L682 (-88.744, 125.8221) -> (-88.7134, 125.8373)
  line L683 (-88.7134, 125.8373) -> (-88.6834, 125.8535)
  line L684 (-88.6834, 125.8535) -> (-88.6539, 125.8708)
  line L685 (-88.6539, 125.8708) -> (-88.625, 125.889)
  line L686 (-88.625, 125.889) -> (-88.5968, 125.9082)
  line L687 (-88.5968, 125.9082) -> (-88.5692, 125.9284)
  line L688 (-88.5692, 125.9284) -> (-88.5424, 125.9495)
  line L689 (-88.5424, 125.9495) -> (-88.5163, 125.9715)
  line L690 (-88.5163, 125.9715) -> (-88.4909, 125.9944)
  line L691 (-88.4909, 125.9944) -> (-88.4664, 126.0181)
  line L692 (-88.4664, 126.0181) -> (-88.4426, 126.0426)
  line L693 (-88.4426, 126.0426) -> (-88.4197, 126.068)
  line L694 (-88.4197, 126.068) -> (-88.3977, 126.0941)
  line L695 (-88.3977, 126.0941) -> (-88.3767, 126.121)
  line L696 (-88.3767, 126.121) -> (-88.3565, 126.1485)
  line L697 (-88.3565, 126.1485) -> (-88.3373, 126.1767)
  line L698 (-88.3373, 126.1767) -> (-88.319, 126.2056)
  line L699 (-88.319, 126.2056) -> (-88.3018, 126.2351)
  line L700 (-88.3018, 126.2351) -> (-88.2856, 126.2651)
  line L701 (-88.2856, 126.2651) -> (-88.2704, 126.2957)
  line L702 (-88.2704, 126.2957) -> (-88.2562, 126.3268)
  line L703 (-88.2562, 126.3268) -> (-88.2432, 126.3583)
  line L704 (-88.2432, 126.3583) -> (-88.2312, 126.3903)
  line L705 (-88.2312, 126.3903) -> (-88.2203, 126.4227)
  line L706 (-88.2203, 126.4227) -> (-88.2105, 126.4554)
  line L707 (-88.2105, 126.4554) -> (-88.2019, 126.4884)
  line L708 (-88.2019, 126.4884) -> (-88.1944, 126.5217)
  line L709 (-88.1944, 126.5217) -> (-88.188, 126.5553)
  line L710 (-88.188, 126.5553) -> (-88.1828, 126.589)
  line L711 (-88.1828, 126.589) -> (-88.1787, 126.6229)
  line L712 (-88.1787, 126.6229) -> (-88.1758, 126.657)
  line L713 (-88.1758, 126.657) -> (-88.174, 126.6911)
  line L714 (-88.174, 126.6911) -> (-88.1735, 126.7252)
  line L715 (-88.1735, 126.7252) -> (-88.1735, 128.7252)
  line L716 (-88.1735, 128.7252) -> (-21.3571, 128.7252)
  line L717 (-21.3571, 128.7252) -> (-21.3571, 126.7252)
  line L718 (-21.3571, 126.7252) -> (-21.3565, 126.6911)
  line L719 (-21.3565, 126.6911) -> (-21.3547, 126.657)
  line L720 (-21.3547, 126.657) -> (-21.3518, 126.6229)
  line L721 (-21.3518, 126.6229) -> (-21.3477, 126.589)
  line L722 (-21.3477, 126.589) -> (-21.3425, 126.5553)
  line L723 (-21.3425, 126.5553) -> (-21.3361, 126.5217)
  line L724 (-21.3361, 126.5217) -> (-21.3286, 126.4884)
  line L725 (-21.3286, 126.4884) -> (-21.32, 126.4554)
  line L726 (-21.32, 126.4554) -> (-21.3102, 126.4227)
  line L727 (-21.3102, 126.4227) -> (-21.2993, 126.3903)
  line L728 (-21.2993, 126.3903) -> (-21.2873, 126.3583)
  line L729 (-21.2873, 126.3583) -> (-21.2743, 126.3268)
  line L730 (-21.2743, 126.3268) -> (-21.2601, 126.2957)
  line L731 (-21.2601, 126.2957) -> (-21.2449, 126.2651)
  line L732 (-21.2449, 126.2651) -> (-21.2287, 126.2351)
  line L733 (-21.2287, 126.2351) -> (-21.2115, 126.2056)
  line L734 (-21.2115, 126.2056) -> (-21.1932, 126.1767)
  line L735 (-21.1932, 126.1767) -> (-21.174, 126.1485)
  line L736 (-21.174, 126.1485) -> (-21.1539, 126.121)
  line L737 (-21.1539, 126.121) -> (-21.1328, 126.0941)
  line L738 (-21.1328, 126.0941) -> (-21.1108, 126.068)
  line L739 (-21.1108, 126.068) -> (-21.0879, 126.0426)
  line L740 (-21.0879, 126.0426) -> (-21.0642, 126.0181)
  line L741 (-21.0642, 126.0181) -> (-21.0396, 125.9944)
  line L742 (-21.0396, 125.9944) -> (-21.0143, 125.9715)
  line L743 (-21.0143, 125.9715) -> (-20.9881, 125.9495)
  line L744 (-20.9881, 125.9495) -> (-20.9613, 125.9284)
  line L745 (-20.9613, 125.9284) -> (-20.9337, 125.9082)
  line L746 (-20.9337, 125.9082) -> (-20.9055, 125.889)
  line L747 (-20.9055, 125.889) -> (-20.8766, 125.8708)
  line L748 (-20.8766, 125.8708) -> (-20.8472, 125.8535)
  line L749 (-20.8472, 125.8535) -> (-20.8171, 125.8373)
  line L750 (-20.8171, 125.8373) -> (-20.7865, 125.8221)
  line L751 (-20.7865, 125.8221) -> (-20.7555, 125.808)
  line L752 (-20.7555, 125.808) -> (-20.7239, 125.7949)
  line L753 (-20.7239, 125.7949) -> (-20.6919, 125.7829)
  line L754 (-20.6919, 125.7829) -> (-20.6596, 125.7721)
  line L755 (-20.6596, 125.7721) -> (-20.6268, 125.7623)
  line L756 (-20.6268, 125.7623) -> (-20.5938, 125.7536)
  line L757 (-20.5938, 125.7536) -> (-20.5605, 125.7461)
  line L758 (-20.5605, 125.7461) -> (-20.527, 125.7397)
  line L759 (-20.527, 125.7397) -> (-20.4932, 125.7345)
  line L760 (-20.4932, 125.7345) -> (-20.4593, 125.7304)
  line L761 (-20.4593, 125.7304) -> (-20.4253, 125.7275)
  line L762 (-20.4253, 125.7275) -> (-20.3912, 125.7258)
  line L763 (-20.3912, 125.7258) -> (-20.3571, 125.7252)
  line L764 (-20.3571, 125.7252) -> (-17.357, 125.7252)
  line L765 (-17.357, 125.7252) -> (-17.3229, 125.7258)
  line L766 (-17.3229, 125.7258) -> (-17.2888, 125.7275)
  line L767 (-17.2888, 125.7275) -> (-17.2548, 125.7304)
  line L768 (-17.2548, 125.7304) -> (-17.2209, 125.7345)
  line L769 (-17.2209, 125.7345) -> (-17.1871, 125.7397)
  line L770 (-17.1871, 125.7397) -> (-17.1536, 125.7461)
  line L771 (-17.1536, 125.7461) -> (-17.1203, 125.7536)
  line L772 (-17.1203, 125.7536) -> (-17.0873, 125.7623)
  line L773 (-17.0873, 125.7623) -> (-17.0545, 125.7721)
  line L774 (-17.0545, 125.7721) -> (-17.0222, 125.7829)
  line L775 (-17.0222, 125.7829) -> (-16.9902, 125.7949)
  line L776 (-16.9902, 125.7949) -> (-16.9586, 125.808)
  line L777 (-16.9586, 125.808) -> (-16.9276, 125.8221)
  line L778 (-16.9276, 125.8221) -> (-16.897, 125.8373)
  line L779 (-16.897, 125.8373) -> (-16.8669, 125.8535)
  line L780 (-16.8669, 125.8535) -> (-16.8375, 125.8708)
  line L781 (-16.8375, 125.8708) -> (-16.8086, 125.889)
  line L782 (-16.8086, 125.889) -> (-16.7804, 125.9082)
  line L783 (-16.7804, 125.9082) -> (-16.7528, 125.9284)
  line L784 (-16.7528, 125.9284) -> (-16.726, 125.9495)
  line L785 (-16.726, 125.9495) -> (-16.6998, 125.9715)
  line L786 (-16.6998, 125.9715) -> (-16.6745, 125.9944)
  line L787 (-16.6745, 125.9944) -> (-16.6499, 126.0181)
  line L788 (-16.6499, 126.0181) -> (-16.6262, 126.0426)
  line L789 (-16.6262, 126.0426) -> (-16.6033, 126.068)
  line L790 (-16.6033, 126.068) -> (-16.5813, 126.0941)
  line L791 (-16.5813, 126.0941) -> (-16.5602, 126.121)
  line L792 (-16.5602, 126.121) -> (-16.5401, 126.1485)
  line L793 (-16.5401, 126.1485) -> (-16.5209, 126.1767)
  line L794 (-16.5209, 126.1767) -> (-16.5026, 126.2056)
  line L795 (-16.5026, 126.2056) -> (-16.4854, 126.2351)
  line L796 (-16.4854, 126.2351) -> (-16.4692, 126.2651)
  line L797 (-16.4692, 126.2651) -> (-16.454, 126.2957)
  line L798 (-16.454, 126.2957) -> (-16.4398, 126.3268)
  line L799 (-16.4398, 126.3268) -> (-16.4268, 126.3583)
  line L800 (-16.4268, 126.3583) -> (-16.4148, 126.3903)
  line L801 (-16.4148, 126.3903) -> (-16.4039, 126.4227)
  line L802 (-16.4039, 126.4227) -> (-16.3941, 126.4554)
  line L803 (-16.3941, 126.4554) -> (-16.3855, 126.4884)
  line L804 (-16.3855, 126.4884) -> (-16.378, 126.5217)
  line L805 (-16.378, 126.5217) -> (-16.3716, 126.5553)
  line L806 (-16.3716, 126.5553) -> (-16.3664, 126.589)
  line L807 (-16.3664, 126.589) -> (-16.3623, 126.6229)
  line L808 (-16.3623, 126.6229) -> (-16.3594, 126.657)
  line L809 (-16.3594, 126.657) -> (-16.3576, 126.6911)
  line L810 (-16.3576, 126.6911) -> (-16.357, 126.7252)
  line L811 (-16.357, 126.7252) -> (-16.3571, 128.7252)
  line L812 (-16.3571, 128.7252) -> (-15.3571, 128.7252)
  spline S11 degree 3 poles (-15.3571, 128.7252) (-14.2525, 128.7252) (-13.3571, 129.6206) (-13.3571, 130.7252) knots 0 0 0 0 1 1 1 1
  line L813 (-15.3571, 128.7252) -> (-14.2525, 128.7252) construction
  line L814 (-14.2525, 128.7252) -> (-13.3571, 129.6206) construction
  line L815 (-13.3571, 129.6206) -> (-13.3571, 130.7252) construction
  line L816 (-91.3571, 75.0912) -> (-93.3571, 75.0912)
  line L817 (-93.3571, 74.7912) -> (-91.3571, 74.7912)
  line L818 (-93.3571, 75.0912) -> (-93.3571, 77.0912)
  line L819 (-93.3571, 77.0912) -> (-94.3571, 77.0912)
  line L820 (-94.3571, 77.0912) -> (-94.3571, 81.0912)
  spline S12 degree 3 poles (-94.3571, 81.0912) (-94.3571, 81.3565) (-94.4624, 81.6108) (-94.6499, 81.7984) knots 0 0 0 0 0.5 0.5 0.5 0.5
  line L821 (-94.3571, 81.0912) -> (-94.3571, 81.3565) construction
  line L822 (-94.3571, 81.3565) -> (-94.4624, 81.6108) construction
  line L823 (-94.4624, 81.6108) -> (-94.6499, 81.7984) construction
  spline S13 degree 3 poles (-94.6499, 81.7984) (-94.650088, 81.798588) (-94.8375, 81.9859) (-95.0918, 82.0912) (-95.3571, 82.0912) knots 0.5 0.5 0.5 0.5 0.50000001 1 1 1 1
  line L824 (-94.6499, 81.7984) -> (-94.6499, 81.7984) construction
  line L825 (-94.6499, 81.7984) -> (-94.8375, 81.9859) construction
  line L826 (-94.8375, 81.9859) -> (-95.0918, 82.0912) construction
  line L827 (-95.0918, 82.0912) -> (-95.3571, 82.0912) construction
  line L828 (-95.3571, 82.0912) -> (-97.3571, 82.0912)
  spline S14 degree 3 poles (-97.3571, 82.0912) (-97.6223, 82.0912) (-97.8766, 81.9859) (-98.0642, 81.7984) knots 0 0 0 0 0.5 0.5 0.5 0.5
  line L829 (-97.3571, 82.0912) -> (-97.6223, 82.0912) construction
  line L830 (-97.6223, 82.0912) -> (-97.8766, 81.9859) construction
  line L831 (-97.8766, 81.9859) -> (-98.0642, 81.7984) construction
  spline S15 degree 3 poles (-98.0642, 81.7984) (-98.064388, 81.798212) (-98.2517, 81.6108) (-98.3571, 81.3565) (-98.3571, 81.0912) knots 0.5 0.5 0.5 0.5 0.50000001 1 1 1 1
  line L832 (-98.0642, 81.7984) -> (-98.0642, 81.7984) construction
  line L833 (-98.0642, 81.7984) -> (-98.2517, 81.6108) construction
  line L834 (-98.2517, 81.6108) -> (-98.3571, 81.3565) construction
  line L835 (-98.3571, 81.3565) -> (-98.3571, 81.0912) construction
  line L836 (-98.3571, 81.0912) -> (-98.3571, 77.0912)